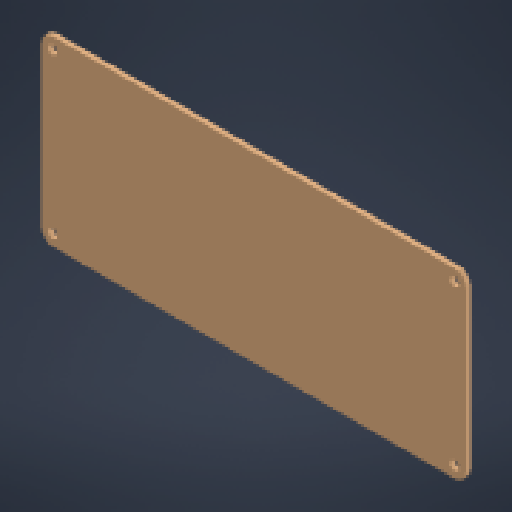
# Autodesk Inventor part: Phased_array
Saved by Autodesk Inventor 2023.4 (Build 274418000, 418)
## iProperties
Created: 2025-09-26
Part Number: Phased_array
Material: Generic
Document SubType Name: Modeling
Designer: Malthe Sennels
Density: 1 g/cm^3
Appearance: Default
Author: Malthe Sennels
Autodesk Inventor part; units mm, degrees
ref_plane "YZ Plane" through (0, 0, 0) normal (1, 0, 0) x (0, 1, 0)
ref_plane "XZ Plane" through (0, 0, 0) normal (0, 1, 0) x (-1, 0, 0)
ref_plane "XY Plane" through (0, 0, 0) normal (0, 0, 1) x (1, 0, 0)
sketch "Sketch1" plane through (0, 0, 0) normal (0, 0, 1) x (1, 0, 0)
  line L0 (-160.1126, 202.6875) -> (-23.9126, 202.6875)
  line L1 (-23.9126, 202.6875) -> (-23.9126, 142.6875)
  line L2 (-23.9126, 142.6875) -> (-163.9126, 142.6875)
  line L3 (-163.9126, 142.6875) -> (-163.9126, 198.8875)
  circle A0 centre (-160.1126, 198.8875) radius 1.5
  arc A1 (-160.1126, 202.6875) -> (-163.9126, 198.8875) centre (-160.1126, 198.8875) ccw
  line L4 (-163.9126, 172.6875) -> (-23.9126, 172.6875) construction
  line L5 (-93.9126, 142.6875) -> (-93.9126, 202.6875) construction
  circle A2 centre (-160.1126, 146.4875) radius 1.5
  circle A3 centre (-27.7126, 198.8875) radius 1.5
  circle A4 centre (-27.7126, 146.4875) radius 1.5
  arc A5 (-163.9126, 146.4875) -> (-160.1126, 142.6875) centre (-160.1126, 146.4875) ccw
  arc A6 (-23.9126, 198.8875) -> (-27.7126, 202.6875) centre (-27.7126, 198.8875) ccw
  arc A7 (-27.7126, 142.6875) -> (-23.9126, 146.4875) centre (-27.7126, 146.4875) ccw
  point P0 (0, 0)
  point P1 (-163.9126, 202.6875)
  dimension "d0" = 60
  dimension "d1" = 140
  dimension "d2" = 3
  dimension "d3" = 3.8
  dimension "d4" = 3.8
  dimension "d5" = 3.8
  constraints: 12 end point, 12 symmetric about line, 8 centre point, 8 point on circle, 4 point on line, 2 midpoint, 2 parallel, 2 perpendicular, 2 tangent, 1 horizontal, 6 other
  measures "d0" distance of L2.end point (-163.913, 202.687)
  measures "d1" distance of L1.end L2.end
  measures "d2" diameter of A0
  measures "d3" distance from line of L0 A0.centre
  measures "d4" distance from line of L3 A0.centre
  measures "d5" radius of A1
extrude "Extrusion1" add sketch "Sketch1" along normal blind 1.6 contours L0 A6 L1 A7 L2 A5 L3 A1
sketch "Sketch2" plane through (0, 0, 0) normal (0, 0, -1) x (-1, 0, 0)
  line L0 (139.9626, 193.3375) -> (107.8626, 193.3375)
  line L1 (107.8626, 193.3375) -> (107.8626, 152.0375) construction
  line L2 (107.8626, 152.0375) -> (139.9626, 152.0375)
  line L3 (139.9626, 152.0375) -> (139.9626, 193.3375)
  line L4 (139.9626, 172.6875) -> (107.8626, 172.6875) construction
  line L5 (117.8626, 176.1875) -> (107.8626, 176.1875)
  line L6 (107.8626, 176.1875) -> (107.8626, 169.1875) construction
  line L7 (107.8626, 169.1875) -> (117.8626, 169.1875)
  line L8 (117.8626, 169.1875) -> (117.8626, 176.1875) construction
  line L9 (117.8626, 176.1875) -> (107.8626, 169.1875) construction
  line L10 (107.8626, 176.1875) -> (117.8626, 169.1875) construction
  line L11 (107.8626, 193.3375) -> (107.8626, 176.1875)
  line L12 (107.8626, 169.1875) -> (107.8626, 152.0375)
  line L13 (93.9126, 174.1875) -> (117.8626, 174.1875)
  line L14 (117.8626, 174.1875) -> (117.8626, 171.1875) construction
  line L15 (117.8626, 171.1875) -> (93.9126, 171.1875)
  line L16 (93.9126, 171.1875) -> (93.9126, 174.1875)
  line L17 (93.9126, 174.1875) -> (117.8626, 171.1875) construction
  line L18 (117.8626, 174.1875) -> (93.9126, 171.1875) construction
  line L19 (117.8626, 174.1875) -> (117.8626, 176.1875)
  line L20 (27.7126, 202.6875) -> (160.1126, 202.6875) projected
  line L21 (160.1126, 142.6875) -> (27.7126, 142.6875) projected
  line L22 (27.7126, 202.6875) -> (160.1126, 202.6875) projected
  line L23 (93.9126, 202.6875) -> (93.9126, 142.6875) construction
  line L24 (163.9126, 198.8875) -> (163.9126, 146.4875) projected
  line L25 (163.9126, 172.6875) -> (23.9126, 172.6875) construction
  line L26 (23.9126, 146.4875) -> (23.9126, 198.8875) projected
  line L27 (123.9126, 193.3375) -> (123.9126, 152.0375) construction
  line L28 (47.8626, 193.3375) -> (79.9626, 193.3375)
  line L29 (79.9626, 193.3375) -> (79.9626, 152.0375) construction
  line L30 (79.9626, 152.0375) -> (47.8626, 152.0375)
  line L31 (47.8626, 152.0375) -> (47.8626, 193.3375)
  line L32 (47.8626, 172.6875) -> (79.9626, 172.6875) construction
  line L33 (69.9626, 176.1875) -> (79.9626, 176.1875)
  line L34 (79.9626, 176.1875) -> (79.9626, 169.1875) construction
  line L35 (79.9626, 169.1875) -> (69.9626, 169.1875)
  line L36 (69.9626, 169.1875) -> (69.9626, 176.1875) construction
  line L37 (69.9626, 176.1875) -> (79.9626, 169.1875) construction
  line L38 (79.9626, 176.1875) -> (69.9626, 169.1875) construction
  line L39 (79.9626, 193.3375) -> (79.9626, 176.1875)
  line L40 (79.9626, 169.1875) -> (79.9626, 152.0375)
  line L41 (93.9126, 174.1875) -> (69.9626, 174.1875)
  line L42 (69.9626, 174.1875) -> (69.9626, 171.1875) construction
  line L43 (69.9626, 171.1875) -> (93.9126, 171.1875)
  line L44 (69.9626, 174.1875) -> (69.9626, 176.1875)
  line L45 (63.9126, 193.3375) -> (63.9126, 152.0375) construction
  line L46 (117.8626, 171.1875) -> (117.8626, 169.1875)
  line L47 (69.9626, 171.1875) -> (69.9626, 169.1875)
  point P0 (0, 0)
  point P1 (112.8626, 172.6875)
  point P2 (105.8876, 172.6875)
  point P3 (93.9126, 172.6875)
  point P4 (74.9626, 172.6875)
  point P5 (81.9376, 172.6875)
  dimension "d8" = 41.3
  dimension "d9" = 32.1
  dimension "d10" = 10
  dimension "d11" = 3
  dimension "d12" = 7
  dimension "d13" = 30
  constraints: 86 end point, 16 symmetric about line, 13 midpoint, 10 point on line, 7 equal length, 4 vertical, 3 horizontal, 3 perpendicular
  measures "d8" distance between parallel lines of L0 L2
  measures "d9" distance of L1.end L2.end
  measures "d10" distance of L6.end L7.end
  measures "d11" distance between parallel lines of L13 L15
  measures "d12" distance between parallel lines of L5 L7
  measures "d13" distance from line of point (93.913, 172.687) L27
extrude "Extrusion2" add sketch "Sketch2" along normal blind 0.035
body "Solid1"
